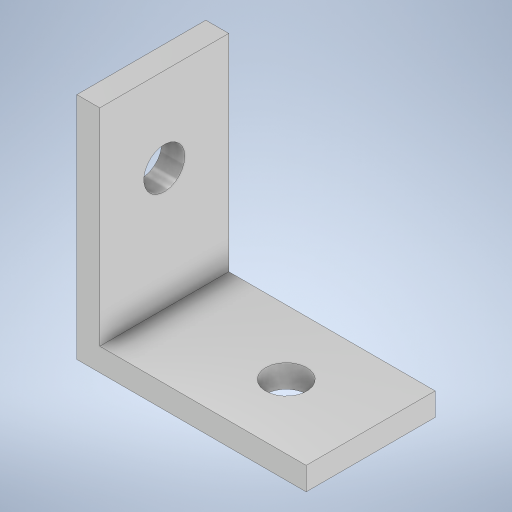
# Autodesk Inventor part: Lbracket
Saved by Autodesk Inventor 2024.3 (Build 283343000, 343)
## iProperties
Created: 2025-01-03
Part Number: Lbracket
Material: Generic
Document SubType Name: Modeling
Designer: email
Density: 1 g/cm^3
Appearance: Default
Author: email
Autodesk Inventor part; units mm, degrees
ref_plane "YZ Plane" through (0, 0, 0) normal (1, 0, 0) x (0, 1, 0)
ref_plane "XZ Plane" through (0, 0, 0) normal (0, 1, 0) x (-1, 0, 0)
ref_plane "XY Plane" through (0, 0, 0) normal (0, 0, 1) x (1, 0, 0)
sketch "Sketch2" plane through (0, 0, 0) normal (0, 0, 1) x (1, 0, 0)
  line L0 (0, 0) -> (40, 0)
  line L1 (40, 0) -> (40, 4)
  line L2 (40, 4) -> (0, 4)
  line L3 (0, 4) -> (0, 0)
  line L4 (0, 0) -> (4, 0)
  line L5 (4, 0) -> (4, 40)
  line L6 (4, 40) -> (0, 40)
  line L7 (0, 40) -> (0, 0)
  point P0 (4, 4)
  point P1 (0, 4)
  dimension "d0" = 40
  dimension "d1" = 40
  dimension "d2" = 4
  dimension "d3" = 4
  constraints: 16 end point, 4 parallel, 2 horizontal, 2 perpendicular
  measures "d0" distance of L0.start L0.end
  measures "d1" distance of L6.end L0.start
  measures "d2" distance of L0.end L1.end
  measures "d3" distance of L5.end L6.end
extrude "Extrusion1" add sketch "Sketch2" along normal blind 22.5
sketch "Sketch3" plane through (0, 0, 0) normal (0, -1, 0) x (1, 0, 0)
  circle A0 centre (25.275, 11.25) radius 5.756
  line L0 (0, 22.5) -> (40, 22.5) projected
  line L1 (0, 0) -> (0, 22.5) projected
  dimension "d6" = 11.25
  dimension "d7" = 25.275
  constraints: 1 centre point
  measures "d6" distance from line of L0 A0.centre
  measures "d7" distance from line of L1 A0.centre
sketch "Sketch4" plane through (0, 0, 0) normal (-1, 0, 0) x (0, 0, 1)
  circle A0 centre (11.25, 25.275) radius 7.6084
  line L0 (22.5, 40) -> (22.5, 0) projected
  line L1 (0, 0) -> (22.5, 0) projected
  line L2 (0, 40) -> (22.5, 40) projected
  dimension "d8" = 11.25
  dimension "d9" = 25.275
  dimension "d24" = 14.725
  constraints: 1 centre point
  measures "d8" distance from line of L0 A0.centre
  measures "d9" distance from line of L1 A0.centre
  measures "d24" distance from line of L2 A0.centre
hole "Hole1" at (0, 25.275, 11.25) direction (1, 0, 0) diameter 7.15 depth 5
hole "Hole2" at (25.275, 0, 11.25) direction (0, 1, 0) diameter 7.15 depth 5
body "Solid1"
